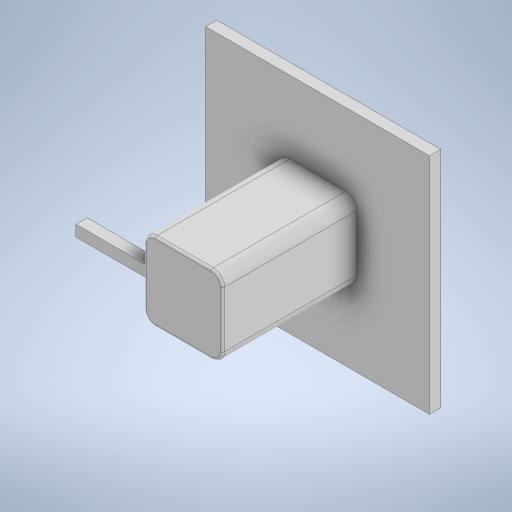
# Autodesk Inventor part: Sign
Saved by Autodesk Inventor 2023 (Build 270158000, 158)
## iProperties
Created: 2022-09-20
Part Number: Sign
Material: Generic
Document SubType Name: Modeling
Designer: benni
Density: 1 g/cm^3
Appearance: Default
Author: benni
Autodesk Inventor part; units mm, degrees
ref_plane "YZ Plane" through (0, 0, 0) normal (1, 0, 0) x (0, 1, 0)
ref_plane "XZ Plane" through (0, 0, 0) normal (0, 1, 0) x (-1, 0, 0)
ref_plane "XY Plane" through (0, 0, 0) normal (0, 0, 1) x (1, 0, 0)
sketch "Sketch1" plane through (0, 0, 0) normal (0, 0, 1) x (1, 0, 0)
  line L0 (-50, -50) -> (50, -50)
  line L1 (50, -50) -> (50, 50)
  line L2 (50, 50) -> (-50, 50)
  line L3 (-50, 50) -> (-50, -50)
  line L4 (-50, -50) -> (50, 50) construction
  line L5 (50, -50) -> (-50, 50) construction
  point P0 (0, 0)
  dimension "d29" = 100
  dimension "d30" = 100
  constraints: 12 end point, 2 midpoint, 2 parallel, 1 horizontal, 1 perpendicular
  measures "d29" distance of L2.end L1.end
  measures "d30" distance of L1.end L0.end
extrude "Extrusion1" add sketch "Sketch1" along normal blind 5
sketch "Sketch2" plane through (0, 0, 5) normal (0, 0, 1) x (1, 0, 0)
  line L0 (-17.5, -17.5) -> (17.5, -17.5)
  line L1 (17.5, -17.5) -> (17.5, 17.5)
  line L2 (17.5, 17.5) -> (-17.5, 17.5)
  line L3 (-17.5, 17.5) -> (-17.5, -17.5)
  line L4 (-17.5, -17.5) -> (17.5, 17.5) construction
  line L5 (17.5, -17.5) -> (-17.5, 17.5) construction
  point P0 (0, 0)
  dimension "d20" = 35
  dimension "d21" = 35
  constraints: 12 end point, 2 midpoint, 2 parallel, 1 horizontal, 1 perpendicular
  measures "d20" distance of L2.end L1.end
  measures "d21" distance of L1.end L0.end
extrude "Extrusion2" add sketch "Sketch2" along normal blind 60
fillet "Fillet1" radius 5 4 edges at (17.5, 17.5, 35) (17.5, -17.5, 35) (-17.5, 17.5, 35) (-17.5, -17.5, 35)
fillet "Fillet2" radius 1 8 edges at (16.0355, 16.0355, 65) (0, 17.5, 65) (-16.0355, 16.0355, 65) (-17.5, 0, 65) (-16.0355, -16.0355, 65) (0, -17.5, 65) (16.0355, -16.0355, 65) (17.5, 0, 65)
sketch "Sketch4" plane through (-17.5, -12.5, 5) normal (-1, 0, 0) x (0, 0, 1)
  line L0 (59, 25) -> (59, 0) projected
  line L1 (59, 0) -> (0, 0) projected
  line L2 (0, 25) -> (59, 25) projected
  line L3 (52.9156, 10) -> (57.9156, 10)
  line L4 (57.9156, 10) -> (57.9156, 15)
  line L5 (57.9156, 15) -> (52.9156, 15)
  line L6 (52.9156, 15) -> (52.9156, 10)
  line L7 (52.9156, 10) -> (57.9156, 15) construction
  line L8 (57.9156, 10) -> (52.9156, 15) construction
  point P0 (-5, 12.5)
  point P1 (55.4156, 12.5)
  dimension "d31" = 5
  dimension "d32" = 5
  constraints: 12 end point, 2 midpoint, 2 parallel, 1 horizontal, 1 perpendicular
  measures "d31" distance of L5.end L4.end
  measures "d32" distance of L4.end L3.end
extrude "Extrusion4" add sketch "Sketch4" along normal up to surface (32.5 mm away)
body "Solid1"
